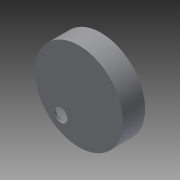
# Autodesk Inventor part: obudowa - czujnik dymu
Saved by Autodesk Inventor 2014 (Build 180170000, 170)
## iProperties
Created: 2018-02-27
Part Number: obudowa - czujnik dymu
Material: Generic
Document SubType Name: Modeling
Designer: HP820
Density: 1 g/cm^3
Appearance: Default
Author: HP820
Autodesk Inventor part; units mm, degrees
ref_plane "YZ Plane" through (0, 0, 0) normal (1, 0, 0) x (0, 1, 0)
ref_plane "XZ Plane" through (0, 0, 0) normal (0, 1, 0) x (-1, 0, 0)
ref_plane "XY Plane" through (0, 0, 0) normal (0, 0, 1) x (1, 0, 0)
sketch "Sketch1" plane through (0, 0, 0) normal (0, 1, 0) x (-1, 0, 0)
  circle A0 centre (0, 0) radius 34
  dimension "d0" = 68
  constraints: 1 centre point, 1 coincident
  measures "d0" diameter of A0
extrude "Extrusion1" add sketch "Sketch1" along normal blind 3
sketch "Sketch2" plane through (0, 3, 0) normal (0, 1, 0) x (1, 0, 0)
  circle A0 centre (0, 0) radius 34 projected
  circle A1 centre (0, 0) radius 31
  dimension "d3" = 62
  constraints: 1 centre point, 1 coincident
  measures "d3" diameter of A1
extrude "Extrusion2" add sketch "Sketch2" along normal blind 14
sketch "Sketch3" plane through (0, 3, 0) normal (0, 1, 0) x (1, 0, 0)
  circle A0 centre (0, 0) radius 31 projected
  circle A1 centre (0, 0) radius 19.5
  line L0 (-19.5, 0) -> (19.5, 0)
  circle A2 centre (-19.5, 0) radius 1.2
  circle A3 centre (-19.5, 0) radius 2.5
  circle A4 centre (19.5, 0) radius 1.2
  circle A5 centre (19.5, 0) radius 2.5
  dimension "d6" = 39
  dimension "d7" = 2.4
  dimension "d8" = 5
  dimension "d9" = 2.4
  dimension "d10" = 5
  constraints: 5 centre point, 5 coincident, 2 end point, 2 point on circle
  measures "d6" diameter of A1
  measures "d7" diameter of A2
  measures "d8" diameter of A3
  measures "d9" diameter of A4
  measures "d10" diameter of A5
extrude "Extrusion3" add sketch "Sketch3" along normal up to surface (14 mm away) contours A4 L0 A5 A1 | A1 A5 A4 | A1 A5 L0 A4 | A3 L0 A2 A1 | A1 A2 A3 | A1 A2 L0 A3
chamfer "Chamfer1" distance 2 angle 45 2 edges at (-22, 3, 0) (17, 3, 0)
sketch "Sketch4" plane through (0, 3, 0) normal (0, 1, 0) x (1, 0, 0)
  circle A0 centre (-13.9417, 19.5241) radius 5
  dimension "d16" = 10
  constraints: 1 centre point
  measures "d16" diameter of A0
extrude "Extrusion4" cut sketch "Sketch4" against normal blind 14
chamfer "Chamfer2" distance 2 angle 45 1 edges at (-18.9417, 3, -19.5241)
sketch "Sketch5" plane through (0, 3, 0) normal (0, 1, 0) x (1, 0, 0)
  line L0 (-8.5812, 13.9919) -> (11.4188, 13.9919)
  line L1 (11.4188, 13.9919) -> (11.4188, -26.0081)
  line L2 (11.4188, -26.0081) -> (-8.5812, -26.0081)
  line L3 (-8.5812, -26.0081) -> (-8.5812, 13.9919)
  circle A0 centre (-5.5812, 10.9919) radius 1.25
  circle A1 centre (-5.5812, 10.9919) radius 3
  circle A2 centre (8.4188, 10.9919) radius 1.25
  circle A3 centre (8.4188, 10.9919) radius 3
  circle A4 centre (8.4188, -23.0081) radius 1.25
  circle A5 centre (8.4188, -23.0081) radius 3
  circle A6 centre (-5.5812, -23.0081) radius 1.25
  circle A7 centre (-5.5812, -23.0081) radius 3
  dimension "d22" = 20
  dimension "d23" = 40
  dimension "d24" = 2.5
  dimension "d25" = 6
  dimension "d26" = 2.5
  dimension "d27" = 6
  dimension "d28" = 2.5
  dimension "d29" = 6
  dimension "d30" = 2.5
  dimension "d31" = 6
  dimension "d32" = 3
  dimension "d33" = 3
  dimension "d34" = 3
  dimension "d35" = 3
  dimension "d36" = 3
  dimension "d37" = 3
  dimension "d38" = 3
  dimension "d39" = 3
  constraints: 8 centre point, 8 end point, 4 coincident, 2 parallel, 1 horizontal, 1 perpendicular
  measures "d22" distance of L1.end L2.end
  measures "d23" distance of L0.end L1.end
  measures "d24" diameter of A0
  measures "d25" diameter of A1
  measures "d26" diameter of A2
  measures "d27" diameter of A3
  measures "d28" diameter of A4
  measures "d29" diameter of A5
  measures "d30" diameter of A6
  measures "d31" diameter of A7
  measures "d32" distance from line of A0.centre L3
  measures "d33" distance from line of L0 A0.centre
  measures "d34" distance from line of L1 A3.centre
  measures "d35" distance from line of L0 A3.centre
  measures "d36" distance from line of L2 A5.centre
  measures "d37" distance from line of L1 A5.centre
  measures "d38" distance from line of A6.centre L2
  measures "d39" distance from line of A7.centre L3
extrude "Extrusion5" add sketch "Sketch5" along normal blind 2 contours A1 | A3 | A7 | A5
sketch "Sketch6" plane through (-5.5812, 3, -10.9919) normal (0, 1, 0) x (1, 0, 0)
  circle A0 centre (0, 0) radius 1.25 projected
  circle A1 centre (0, 0) radius 1.25 projected
  circle A2 centre (14, 0) radius 1.25 projected
  circle A3 centre (14, -34) radius 1.25 projected
  circle A4 centre (0, -34) radius 1.25 projected
  point P0 (5.5812, -10.9919)
extrude "Extrusion6" cut sketch "Sketch6" against normal blind 2
chamfer "Chamfer3" distance 0.5 angle 45 4 edges at (-6.8312, 5, -10.9919) (7.1688, 5, -10.9919) (-6.8312, 5, 23.0081) (7.1688, 5, 23.0081)
body "Solid1"
